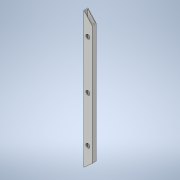
# Autodesk Inventor part: AngleBrace.ver1-1111-2020
Saved by Autodesk Inventor 2021 (Build 250183000, 183)
## iProperties
Created: 2020-01-19
Part Number: AngleBrace.ver1-1111-2020
Material: Generic
Document SubType Name: Modeling
Designer: JMHal
Density: 1 g/cm^3
Appearance: Default
Author: JMHal
Autodesk Inventor part; units mm, degrees
ref_plane "YZ Plane" through (0, 0, 0) normal (1, 0, 0) x (0, 1, 0)
ref_plane "XZ Plane" through (0, 0, 0) normal (0, 1, 0) x (-1, 0, 0)
ref_plane "XY Plane" through (0, 0, 0) normal (0, 0, 1) x (1, 0, 0)
sketch "Sketch1" plane through (0, 0, 0) normal (0, 1, 0) x (-1, 0, 0)
  line L0 (0, 0) -> (50.8, 0)
  line L1 (50.8, 0) -> (50.8, -25.4)
  line L2 (50.8, -25.4) -> (0, -25.4)
  line L3 (0, -25.4) -> (0, 0)
  line L4 (47.625, -22.225) -> (47.625, -3.175)
  line L5 (47.625, -3.175) -> (3.175, -3.175)
  line L6 (3.175, -3.175) -> (3.175, -22.225)
  line L7 (3.175, -22.225) -> (47.625, -22.225)
  dimension "d0" = 50.8
  dimension "d1" = 25.4
  dimension "d2" = 3.175
  constraints: 16 end point, 4 parallel, 2 perpendicular, 1 horizontal, 3 other
  measures "d0" distance of L1.end L2.end
  measures "d1" distance of L0.end L1.end
  measures "d2" distance between parallel lines of L1 L4
extrude "Extrusion1" add sketch "Sketch1" along normal blind 886.206
sketch "Sketch2" plane through (-50.8, 0, 0) normal (0, 0, 1) x (1, 0, 0)
  line L0 (50.8, 0) -> (0, 0) projected
  line L1 (50.8, 0) -> (50.8, 886.206) projected
  line L2 (0, 886.206) -> (50.8, 886.206) projected
  line L3 (0, 0) -> (0, 886.206) projected
  line L4 (0, 0) -> (50.8, 0) projected
  line L5 (50.8, 0) -> (0, 56.4191)
  line L6 (0, 56.4191) -> (50.8, 56.4191)
  line L7 (50.8, 56.4191) -> (50.8, 0)
  line L8 (50.8, 0) -> (0, 0)
  line L9 (0, 0) -> (0, 56.4191)
  line L10 (0, 56.4191) -> (50.8, 0)
  line L11 (0, 56.4191) -> (21.859, 0)
  line L12 (47.625, 0) -> (3.175, 0) projected
  dimension "d5" = 48
  constraints: 14 end point, 2 parallel, 2 point on line, 1 horizontal, 1 perpendicular
  measures "d5" angle of L5 L0
extrude "Extrusion2" cut sketch "Sketch2" against normal blind 914.4 contours L0 L11 L5 | L11 L0 L3
sketch "Sketch3" plane through (-50.8, 886.206, 0) normal (0, 0, 1) x (1, 0, 0)
  line L0 (0, -829.7869) -> (50.8, -886.206) projected
  line L1 (50.8, -886.206) -> (50.8, 0) projected
  line L2 (0, 0) -> (50.8, 0) projected
  line L3 (0, -829.7869) -> (0, 0) projected
  line L4 (0, -829.7869) -> (50.8, -886.206) projected
  line L5 (0, -829.7869) -> (50.8, -784.0464)
  line L6 (50.8, -886.206) -> (50.8, 0) projected
  line L7 (0, -829.7869) -> (0, 0) projected
  line L8 (50.8, -886.206) -> (0, -886.206)
  line L9 (0, -886.206) -> (0, -923.3654)
  line L10 (0, -923.3654) -> (50.8, -923.3654)
  line L11 (50.8, -923.3654) -> (50.8, -886.206)
  dimension "d8" = 90
  constraints: 10 end point, 4 point on line, 2 parallel, 1 horizontal, 1 perpendicular
  measures "d8" angle of L0 L5
extrude "Extrusion3" cut sketch "Sketch3" against normal blind 25.4 contours L5 L1 L0
sketch "Sketch4" plane through (-50.8, 886.206, 0) normal (0, 0, 1) x (1, 0, 0)
  line L0 (0, -829.7869) -> (50.8, -784.0464) projected
  line L1 (50.8, -784.0464) -> (50.8, 0) projected
  line L2 (0, 0) -> (50.8, 0) projected
  line L3 (0, -829.7869) -> (0, 0) projected
  line L4 (0, 0) -> (50.8, 0) projected
  line L5 (0, 0) -> (50.8, 0)
  line L6 (50.8, 0) -> (50.8, -221.7928)
  line L7 (50.8, -221.7928) -> (0, -221.7928)
  line L8 (0, -221.7928) -> (0, 0)
  line L9 (0, -829.7869) -> (0, 0) projected
  line L10 (0, 0) -> (50.8, -56.4191)
  line L11 (50.8, 0) -> (0, 0)
  line L12 (0, 0) -> (0, -56.4191)
  line L13 (0, -56.4191) -> (50.8, -56.4191)
  line L14 (50.8, -56.4191) -> (50.8, 0)
  point P0 (50.8, -886.206)
  dimension "d11" = 221.7928
  dimension "d12" = 48
  dimension "d13" = 56.4191
  constraints: 18 end point, 4 parallel, 3 point on line, 2 horizontal, 2 perpendicular
  measures "d11" distance between parallel lines of L7 L2
  measures "d12" angle of L2 L10
  measures "d13" distance between parallel lines of L13 L2
extrude "Extrusion4" cut sketch "Sketch4" against normal blind 25.4 contours L10 L2 L1
sketch "Sketch8" plane through (-50.8, 56.4191, 0) normal (0, 0, 1) x (1, 0, 0)
  circle A0 centre (25.4, 702.7869) radius 12.7
  line L0 (0, 0) -> (0, 829.7869) projected
  circle A1 centre (25.4, 127) radius 12.7
  circle A2 centre (25.4, 406.4) radius 12.7
  point P0 (50.8, -56.4191)
  dimension "d24" = 25.4
  dimension "d25" = 25.4
  dimension "d26" = 127
  dimension "d27" = 25.4
  dimension "d28" = 25.4
  dimension "d29" = 127
  dimension "d32" = 25.4
  dimension "d37" = 279.4
  constraints: 3 centre point
  measures "d24" diameter of A0
  measures "d25" distance from line of A0.centre L0
  measures "d26" vertical distance of A0.centre L0.end
  measures "d27" diameter of A1
  measures "d28" distance from line of A1.centre L0
  measures "d29" vertical distance of A1.centre L0.start
  measures "d32" diameter of A2
  measures "d37" distance of A2.centre A1.centre
extrude "Extrusion8" cut sketch "Sketch8" against normal blind 25.4
body "Solid1"
